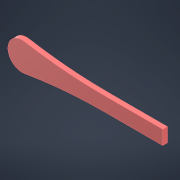
# Autodesk Inventor part: Рычаг_2
Saved by Autodesk Inventor 2021.2 (Build 252289000, 289)
## iProperties
Created: 2021-05-30
Part Number: Рычаг_2
Material: Типовые
Document SubType Name: Modeling
Designer: Admin
Density: 1 g/cm^3
Appearance: Гладкий - красный
Mass: 15.6569 g
Surface Area: 80.7764 cm^2
Volume: 15.6569 cm^3
Author: Admin
Autodesk Inventor part; units mm, degrees
ref_plane "YZ Plane" through (0, 0, 0) normal (1, 0, 0) x (0, 1, 0)
ref_plane "XZ Plane" through (0, 0, 0) normal (0, 1, 0) x (-1, 0, 0)
ref_plane "XY Plane" through (0, 0, 0) normal (0, 0, 1) x (1, 0, 0)
sketch "Эскиз1" plane through (0, 0, 0) normal (0, 0, 1) x (1, 0, 0)
  arc A0 (2.5506, 14.7816) -> (2.5506, -14.7816) centre (0, 0) ccw
  line L0 (87.5714, 7.5) -> (150, 7.5)
  line L1 (150, 7.5) -> (150, -7.5)
  line L2 (150, -7.5) -> (87.5714, -7.5)
  arc A1 (2.5506, 14.7816) -> (87.5714, 7.5) centre (87.5714, 507.5) ccw
  arc A2 (87.5714, -7.5) -> (2.5506, -14.7816) centre (87.5714, -507.5) ccw
  point P0 (12.9904, 7.5)
  point P1 (12.9904, -7.5)
  point P2 (12.9904, 7.5)
  point P3 (12.9904, -7.5)
  dimension "d0" = 30
  dimension "d1" = 150
  dimension "d13" = 15
  dimension "d14" = 7.5
  dimension "d19" = 500
  constraints: 10 point on circle, 6 end point, 4 point on line, 4 tangent, 3 centre point, 2 horizontal, 1 coincident, 1 equal radius, 1 vertical
  measures "d0" diameter of A0
  measures "d1" distance from line of L1 point (0, 0)
  measures "d13" distance between parallel lines of L2 L0
  measures "d14" distance from line of point (0, 0) L2
  measures "d19" radius of A1
extrude "Выдавливание1" add sketch "Эскиз1" along normal blind 5
sketch "Эскиз2" plane through (0, 0, 5) normal (0, 0, 1) x (1, 0, 0)
  arc A0 (2.5506, 14.7816) -> (2.5506, -14.7816) centre (0, 0) ccw projected
  circle A1 centre (0, 0) radius 5
  point P0 (7.7262, 12.8571)
  point P1 (7.7262, -12.8571)
  dimension "d16" = 10
  constraints: 2 coincident, 1 centre point
  measures "d16" diameter of A1
extrude "Выдавливание2" add sketch "Эскиз2" against normal blind 10
equation "\"d14\" = 0.5 * d13"
